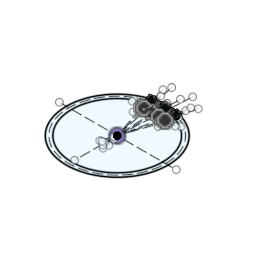
sphere2_top_holder v2 (Autodesk Fusion 360 design; units mm, degrees)
Autodesk Fusion 360 part; units mm, degrees
sketch "Skizze1" plane through (0, 0, 0) normal (0, 0, 1) x (1, 0, 0)
  line L0 (-91.6234, 0) -> (93.3902, 0) construction
  line L1 (0, 100) -> (0, -67.3304) construction
  circle A0 centre (0, 0) radius 80.5
  circle A1 centre (0, 0) radius 76.5 construction
  circle A2 centre (0, 0) radius 72
  line L2 (-20, 88.8476) -> (-20, 45) construction
  line L3 (20, 88.3894) -> (20, 45) construction
  line L4 (-26.8535, 99.1422) -> (2.0736, -7.6557) construction
  line L5 (27.3365, 100.9255) -> (-1.1615, -4.2882) construction
  line L6 (-17.5848, 71.4372) -> (-16.7121, 74.7299)
  line L7 (-16.7121, 74.7299) -> (-19.1273, 77.132)
  line L8 (-19.1273, 77.132) -> (-22.4152, 76.2415)
  line L9 (-22.4152, 76.2415) -> (-23.2879, 72.9488)
  line L10 (-23.2879, 72.9488) -> (-20.8727, 70.5467)
  line L11 (-20.8727, 70.5467) -> (-17.5848, 71.4372)
  line L12 (1.7032, 73.55) -> (3.4064, 76.5)
  line L13 (3.4064, 76.5) -> (1.7032, 79.45)
  line L14 (1.7032, 79.45) -> (-1.7032, 79.45)
  line L15 (-1.7032, 79.45) -> (-3.4064, 76.5)
  line L16 (-3.4064, 76.5) -> (-1.7032, 73.55)
  line L17 (-1.7032, 73.55) -> (1.7032, 73.55)
  line L18 (20.8727, 70.5467) -> (23.2879, 72.9488)
  line L19 (23.2879, 72.9488) -> (22.4152, 76.2415)
  line L20 (22.4152, 76.2415) -> (19.1273, 77.132)
  line L21 (19.1273, 77.132) -> (16.7121, 74.7299)
  line L22 (16.7121, 74.7299) -> (17.5848, 71.4372)
  line L23 (17.5848, 71.4372) -> (20.8727, 70.5467)
  line L24 (-25.543, 76.3401) -> (6.6157, -19.7722) construction
  line L25 (25.543, 76.3401) -> (-6.9044, -20.6352) construction
  line L26 (-36.7956, 63) -> (38.2692, 63) construction
  line L27 (-3.75, 63) -> (-3.75, 59)
  line L28 (3.75, 63) -> (3.75, 59)
  line L29 (-35.5034, 59) -> (32.8477, 59) construction
  line L30 (6.75, 56) -> (16.5776, 56)
  line L31 (-6.75, 56) -> (-16.5776, 56)
  arc A3 (-6.75, 56) -> (-3.75, 59) centre (-6.75, 59) ccw
  arc A4 (3.75, 59) -> (6.75, 56) centre (6.75, 59) ccw
  line L32 (25.543, 76.3401) -> (19.4226, 58.0481)
  line L33 (-25.543, 76.3401) -> (-19.4226, 58.0481)
  arc A5 (3.75, 63) -> (-3.75, 63) centre (0, 63) ccw
  circle A6 centre (-20, 73.8394) radius 1.75
  circle A7 centre (0, 76.5) radius 1.75
  circle A8 centre (20, 73.8394) radius 1.75
  line L34 (-22.9104, 109.1387) -> (5.9662, -28.4213) construction
  line L35 (6.5087, 112.8815) -> (-1.1074, -19.2056) construction
  line L36 (-4.8385, 83.9155) -> (1.4083, -24.4243) construction
  line L37 (20.2185, 96.3153) -> (-4.1334, -19.6904) construction
  line L38 (16.5381, 78.7829) -> (14.7919, 70.4642)
  line L39 (4.6339, 80.3665) -> (4.1446, 71.8806)
  line L40 (-4.6339, 80.3665) -> (-4.1446, 71.8806)
  line L41 (-16.5381, 78.7829) -> (-14.7919, 70.4642)
  arc A9 (-19.4226, 58.0481) -> (-16.5776, 56) centre (-16.5776, 59) ccw
  arc A10 (16.5776, 56) -> (19.4226, 58.0481) centre (16.5776, 59) ccw
  point P0 (-20, 73.8394)
  point P1 (0, 76.5)
  point P2 (20, 73.8394)
  point P3 (-20, 73.8394)
  point P4 (0, 76.5)
  point P5 (20, 73.8394)
  point P6 (0, 63)
  point P7 (-6.75, 59)
  point P8 (6.75, 59)
  point P9 (23.6676, 73.7977)
  point P10 (-16.5776, 56)
  point P11 (-19.4226, 58.0481)
  point P12 (-16.5776, 59)
  point P13 (16.5776, 56)
  point P14 (19.4226, 58.0481)
  point P15 (16.5776, 59)
  dimension "d1" = 161
  dimension "d2" = 153
  dimension "d3" = 144
  dimension "d4" = 20
  dimension "d5" = 20
  dimension "d6" = 5.9
  dimension "d7" = 5.9
  dimension "d8" = 5.9
  dimension "d9" = 18.5
  dimension "d10" = 18.5
  dimension "d11" = 63
  dimension "d13" = 4
  dimension "d24" = 3.5
  dimension "d25" = 3.5
  dimension "d26" = 3.5
  dimension "d33" = 3.3
  dimension "d34" = 3.3
  dimension "d35" = 3.3
  dimension "d36" = 3.3
  constraint horizontal L0
  constraint coincident A0.centre L0
  constraint vertical L1
  constraint coincident A0.centre L1
  constraint coincident A0.centre A1.centre
  constraint vertical L2
  constraint vertical L3
  constraint coincident A1 P3
  constraint coincident L2 P3
  constraint coincident A1 P4
  constraint coincident L1 P4
  constraint coincident L3 P5
  constraint coincident A1 P5
  constraint coincident A0.centre L4
  constraint coincident A0.centre L5
  constraint coincident P5 L5
  constraint coincident P3 L4
  constraint coincident P3 P0
  constraint coincident P4 P1
  constraint coincident P5 P2
  constraint coincident A0.centre L25
  constraint coincident A0.centre L24
  constraint coincident A0 L25.start
  constraint coincident A0 L24.start
  constraint horizontal L26
  constraint coincident L1 P6
  constraint coincident L26 P6
  constraint perpendicular L26 L27
  constraint perpendicular L26 L28
  constraint horizontal L29
  constraint perpendicular L3 L30
  constraint perpendicular L2 L31
  constraint coincident P7 A3.centre
  constraint coincident P8 A4.centre
  constraint coincident L24.start L33.start
  constraint coincident L25.start L32.start
  constraint coincident P6 A5.centre
  constraint coincident A0.centre L34
  constraint coincident A0.centre L35
  constraint coincident A0.centre L36
  constraint coincident A0.centre L37
  constraint coincident A2 L41.end
  constraint coincident L34 L41.end
  constraint coincident A0 L41.start
  constraint coincident L34 L41.start
  constraint coincident A0 L40.start
  constraint coincident L36 L40.start
  constraint coincident L36 L40.end
  constraint coincident A2 L40.end
  constraint coincident A2 L39.end
  constraint coincident L35 L39.end
  constraint coincident L35 L39.start
  constraint coincident A0 L39.start
  constraint coincident A0 L38.start
  constraint coincident L37 L38.end
  constraint coincident A2 L38.end
  constraint coincident L37 L38.start
  constraint coincident L24 P11
  constraint coincident L25 P14
  constraint coincident L31 P10
  constraint coincident P10 L31.end
  constraint coincident P11 L33.end
  constraint coincident P12 A9.centre
  constraint coincident L30 P13
  constraint coincident P14 L32.end
  constraint coincident P15 A10.centre
  measures "d1" diameter of A0
  measures "d2" diameter of A1
  measures "d3" diameter of A2
  measures "d4" distance of L1 L2
  measures "d5" distance of L1 L3
  measures "d6" distance of L8 L11
  measures "d7" distance of L20 L23
  measures "d8" distance of L14 L17
  measures "d9" angle of L1 L24
  measures "d10" angle of L1 L25
  measures "d11" distance of L0 L26
  measures "d13" distance of L26 L29
  measures "d24" diameter of A8
  measures "d25" diameter of A7
  measures "d26" diameter of A6
  measures "d33" angle of L4 L34
  measures "d34" angle of L1 L36
  measures "d35" angle of L1 L35
  measures "d36" angle of L5 L37
extrude "Extrusion1" add sketch "Skizze1" along normal blind 2 contours A0 A2 L32 L38 | A0 A2 L33 L41 | A0 A2 L38 L39 | A2 L27 L28 L30 L31 A3 A4 L32 L33 A5 A9 A10 | A0 A2 L40 L41 | A0 A2 L39 L40 | L6 L7 L8 L9 L10 L11 | L12 L13 L14 L15 L16 L17 | L18 L19 L20 L21 L22 L23 | A6 | A7 | A8 picked at (-11.7065, 63.1547)
extrude "Extrusion2" add sketch "Skizze1" along normal blind 5.8 contours A0 A2 L32 L38 | A0 A2 L33 L41 | A0 A2 L39 L40 | L6 L7 L8 L9 L10 L11 | L12 L13 L14 L15 L16 L17 | L18 L19 L20 L21 L22 L23 | A6 | A7 | A8
extrude "Extrusion3" cut sketch "Skizze1" along normal blind 20 contours A6 | A7 | A8
extrude "Extrusion4" cut sketch "Skizze1" along normal blind 4.8 contours L6 L7 L8 L9 L10 L11 | L12 L13 L14 L15 L16 L17 | L18 L19 L20 L21 L22 L23
extrude "Extrusion5" add sketch "Skizze1" along normal blind 2 contours L6 L7 L8 L9 L10 L11 | L12 L13 L14 L15 L16 L17 | L18 L19 L20 L21 L22 L23
